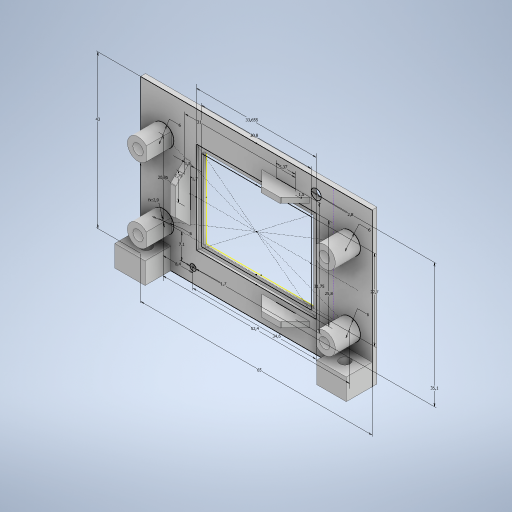
# Autodesk Inventor part: clamp
Saved by Autodesk Inventor 2024 (Build 280153000, 153)
## iProperties
Created: 2024-09-23
Part Number: clamp
Material: Generic
Document SubType Name: Modeling
Designer: PC
Density: 1 g/cm^3
Appearance: Default
Author: PC
Autodesk Inventor part; units mm, degrees
ref_plane "YZ Plane" through (0, 0, 0) normal (1, 0, 0) x (0, 1, 0)
ref_plane "XZ Plane" through (0, 0, 0) normal (0, 1, 0) x (-1, 0, 0)
ref_plane "XY Plane" through (0, 0, 0) normal (0, 0, 1) x (1, 0, 0)
sketch "Sketch1" plane through (0, 0, 0) normal (0, 0, 1) x (1, 0, 0)
  circle A0 centre (0, 0) radius 1.45
  line L0 (0, 0) -> (29.0858, 0) construction
  line L1 (0, 0) -> (0, 12.0151) construction
  circle A1 centre (52.4, 0) radius 1.45
  circle A2 centre (0, 20.95) radius 1.45
  circle A3 centre (52.4, 20.95) radius 1.45
  line L2 (9.3725, 23.375) -> (43.0275, 23.375)
  line L3 (43.0275, 23.375) -> (43.0275, -2.425)
  line L4 (43.0275, -2.425) -> (9.3725, -2.425)
  line L5 (9.3725, -2.425) -> (9.3725, 23.375)
  line L6 (0, 0) -> (52.4, 0) construction
  line L7 (0, 0) -> (0, 20.95) construction
  line L8 (31.8025, 26.35) -> (37.1725, 26.35)
  line L9 (37.1725, 26.35) -> (37.1725, 24.85)
  line L10 (37.1725, 24.85) -> (31.8025, 24.85)
  line L11 (31.8025, 24.85) -> (31.8025, 26.35)
  line L12 (0, 10.475) -> (54.8086, 10.475) construction
  line L13 (31.8025, -5.4) -> (37.1725, -5.4)
  line L14 (37.1725, -5.4) -> (37.1725, -3.9)
  line L15 (37.1725, -3.9) -> (31.8025, -3.9)
  line L16 (31.8025, -3.9) -> (31.8025, -5.4)
  line L17 (6.1725, 14.35) -> (7.6725, 14.35)
  line L18 (7.6725, 14.35) -> (7.6725, 6.6)
  line L19 (7.6725, 6.6) -> (6.1725, 6.6)
  line L20 (6.1725, 6.6) -> (6.1725, 14.35)
  line L21 (-6.3, 31.975) -> (58.7, 31.975)
  line L22 (58.7, 31.975) -> (58.7, -11.025)
  line L23 (58.7, -11.025) -> (-6.3, -11.025)
  line L24 (-6.3, -11.025) -> (-6.3, 31.975)
  line L25 (10.8, 21.825) -> (41.6, 21.825)
  line L26 (41.6, 21.825) -> (41.6, -0.875)
  line L27 (41.6, -0.875) -> (10.8, -0.875)
  line L28 (10.8, -0.875) -> (10.8, 21.825)
  line L29 (9.3725, -2.425) -> (43.0275, 23.375) construction
  line L30 (9.3725, 23.375) -> (43.0275, -2.425) construction
  circle A4 centre (0, 0) radius 3
  circle A5 centre (0, 20.95) radius 3
  circle A6 centre (52.4, 20.95) radius 3
  circle A7 centre (52.4, 0) radius 3
  line L31 (0, 0) -> (52.4, 20.95) construction
  line L32 (0, 20.95) -> (52.4, 0) construction
  circle A8 centre (8.4, -7.1) radius 0.85
  circle A9 centre (43, 28) radius 1.4
  point P0 (9.3725, 10.475)
  point P1 (26.2, 0)
  point P2 (26.2, -2.425)
  point P3 (7.6725, 10.475)
  point P4 (37.1725, 25.6)
  point P5 (26.2, 10.475)
  point P6 (26.2, 21.825)
  point P7 (26.2, 10.475)
  point P8 (41.6, 10.475)
  point P9 (-6.3, 10.475)
  point P10 (26.2, 31.975)
  dimension "d0" = 2.9
  dimension "d3" = 52.4
  dimension "d6" = 20.95
  dimension "d9" = 33.655
  dimension "d10" = 25.8
  dimension "d11" = 5.37
  dimension "d12" = 1.5
  dimension "d15" = 7.75
  dimension "d16" = 31.75
  dimension "d17" = 31
  dimension "d18" = 1.5
  dimension "d19" = 1.7
  dimension "d20" = 30.8
  dimension "d21" = 22.7
  dimension "d22" = 43
  dimension "d23" = 65
  dimension "d31" = 6
  dimension "d32" = 6
  dimension "d33" = 6
  dimension "d34" = 6
  dimension "d50" = 7.1
  dimension "d51" = 34.6
  dimension "d52" = 8.4
  dimension "d53" = 1.7
  dimension "d54" = 2.8
  dimension "d55" = 35.1
  constraints: 66 end point, 12 midpoint, 10 centre point, 10 parallel, 9 horizontal, 5 coincident, 5 perpendicular, 4 symmetric about line, 3 horizontal alignment, 3 vertical, 3 vertical alignment, 1 point on line, 6 other
  measures "d0" diameter of A0
  measures "d3" distance of L0.start L6.end
  measures "d6" distance of L0.start L7.end
  measures "d9" distance of L2.start L2.end
  measures "d10" distance of L2.end L3.end
  measures "d11" distance of L8.start L8.end
  measures "d12" distance of L8.end L9.end
  measures "d15" distance of L19.end L17.start
  measures "d16" distance between parallel lines of L13 L8
  measures "d17" distance from line of L20 point (37.173, 25.6)
  measures "d18" distance of L17.start L17.end
  measures "d19" distance between parallel lines of L5 L18
  measures "d20" distance of L25.start L25.end
  measures "d21" distance of L25.end L26.end
  measures "d22" distance of L23.end L21.start
  measures "d23" distance between parallel lines of L22 L24
  measures "d31" diameter of A4
  measures "d32" diameter of A5
  measures "d33" diameter of A6
  measures "d34" diameter of A7
  measures "d50" vertical distance of A8.centre point (0, 0)
  measures "d51" horizontal distance of A9.centre A8.centre
  measures "d52" horizontal distance of point (0, 0) A8.centre
  measures "d53" diameter of A8
  measures "d54" diameter of A9
  measures "d55" vertical distance of A8.centre A9.centre
extrude "Extrusion1" add sketch "Sketch1" against normal blind 1.4 contours L8 L9 L10 L11 | L16 L15 L14 L13 | L17 L18 L19 L20 | L21 L22 L23 L24 | A4 | A5 | A6 | A7 | A8 | A9
extrude "Extrusion2" add sketch "Sketch1" along normal blind 4.2 contours L8 L9 L10 L11 | L16 L15 L14 L13 | L17 L18 L19 L20
extrude "Extrusion3" add sketch "Sketch1" along normal blind 7 contours A4 | A5 | A6 | A7
sketch "Sketch3" plane through (0, 20.95, 7) normal (0, 0, 1) x (1, 0, 0)
  line L0 (2.3, 3.2266) -> (50.1, 3.2266)
  line L1 (50.1, 3.2266) -> (50.1, -23.7734)
  line L2 (50.1, -23.7734) -> (2.3, -23.7734)
  line L3 (2.3, -23.7734) -> (2.3, 3.2266)
  circle A0 centre (0, 0) radius 3 projected
  circle A1 centre (52.4, 0) radius 3 projected
  line L4 (2.3, -23.7734) -> (50.1, 3.2266) construction
  line L5 (2.3, 3.2266) -> (50.1, -23.7734) construction
  line L6 (9.3725, 2.425) -> (43.0275, 2.425) construction
  line L7 (4.5388, -3.9941) -> (9.4225, -3.9941)
  line L8 (9.4225, -3.9941) -> (9.4225, -17.6824)
  line L9 (9.4225, -17.6824) -> (4.5388, -17.6824)
  line L10 (4.5388, -17.6824) -> (4.5388, -3.9941)
  point P0 (0, -20.95)
  point P1 (26.2, -10.2734)
  point P2 (26.2, 2.425)
  point P3 (2.3, 1.9261)
  point P4 (2.3, -1.9261)
  point P5 (50.1, -1.9261)
  point P6 (50.1, 1.9261)
  dimension "d37" = 47.8
  dimension "d40" = 27
  constraints: 20 end point, 4 parallel, 2 horizontal, 2 midpoint, 2 perpendicular, 1 vertical alignment
  measures "d37" distance of L0.start L0.end
  measures "d40" distance between parallel lines of L2 L0
extrude "Extrusion4" cut sketch "Sketch3" against normal up to surface (7 mm away) contours L0 L1 A1 L2 L3 A0 | A0 L3 | L1 A1 picked at (2.4273, 0.4482) picked at (49.8935, -0.2303)
extrude "Extrusion5" add sketch "Sketch1" against normal blind 1.4 contours L2 L3 L4 L5
extrude "Extrusion6" cut sketch "Sketch1" against normal blind 0.7 contours L2 L3 L4 L5
sketch "Sketch5" plane through (0, 0, 0) normal (0, 0, 1) x (1, 0, 0)
  line L0 (58.7, -11.025) -> (-6.3, -11.025) construction
  line L1 (47.9657, -11.025) -> (47.9657, 31.975) construction
  line L2 (-6.3, 31.975) -> (58.7, 31.975) construction
  point P0 (0, 0)
  constraints: 2 end point, 2 point on line, 1 vertical
sketch "Sketch2" plane through (-6.3, -11.025, 0) normal (0, -1, 0) x (1, 0, 0)
  circle A0 centre (60.9, 3.5) radius 1.45
  circle A1 centre (5.1, 3.5) radius 1.5013
  line L0 (0, 0) -> (65, 0) projected
  line L1 (5.1, 3.5) -> (60.9, 3.5) construction
  line L2 (65, 0) -> (56.7123, 0)
  line L3 (56.7123, 0) -> (56.7123, 7.2261)
  line L4 (56.7123, 7.2261) -> (65, 7.2261)
  line L5 (65, 7.2261) -> (65, 0)
  line L6 (8.4882, 7.2261) -> (0, 7.2261)
  line L7 (0, 7.2261) -> (0, 0)
  line L8 (0, 0) -> (8.4882, 0)
  line L9 (8.4882, 0) -> (8.4882, 7.2261)
  point P0 (6.3, 0)
  point P1 (56.4, 7)
  dimension "d28" = 2.9
  dimension "d29" = 55.8
  dimension "d30" = 3.5
  dimension "d47" = 4.5
  constraints: 18 end point, 4 parallel, 3 horizontal, 2 centre point, 2 perpendicular, 1 point on line
  measures "d28" diameter of A0
  measures "d29" distance of L1.end L1.start
  measures "d30" distance from line of L0 L1.start
  measures "d47" horizontal distance of L1.end point (56.4, 7)
sketch "Sketch4" plane through (0, 0, -1.4) normal (0, 0, -1) x (-1, 0, 0)
  line L0 (-7.1929, 23.3228) -> (-45.2071, 23.3228)
  line L1 (-45.2071, 23.3228) -> (-45.2071, -2.3728)
  line L2 (-45.2071, -2.3728) -> (-7.1929, -2.3728)
  line L3 (-7.1929, -2.3728) -> (-7.1929, 23.3228)
  line L4 (-2.8715, 28.8309) -> (-49.5285, 28.8309)
  line L5 (-49.5285, 28.8309) -> (-49.5285, -7.8809)
  line L6 (-49.5285, -7.8809) -> (-2.8715, -7.8809)
  line L7 (-2.8715, -7.8809) -> (-2.8715, 28.8309)
  line L8 (-10.8, -0.875) -> (-41.6, -0.875) projected
  line L9 (-10.8, 21.825) -> (-10.8, -0.875) projected
  point P0 (0, 0)
  point P1 (-26.2, -2.3728)
  point P2 (-26.2, -0.875)
  point P3 (-10.8, 10.475)
  point P4 (-7.1929, 10.475)
  point P5 (-2.8715, 10.475)
  point P6 (-26.2, -7.8809)
  point P7 (-26.2, -0.875)
  constraints: 16 end point, 7 midpoint, 4 parallel, 3 vertical alignment, 2 horizontal, 2 horizontal alignment, 2 perpendicular
extrude "Extrusion7" add sketch "Sketch2" against normal blind 6
extrude "Extrusion8" cut sketch "Sketch1" against normal through all contours A8 | A9
chamfer "Chamfer1" distance 4 angle 45 6 edges at (6.9225, 14.35, 0) (6.9225, 6.6, 0) (31.8025, -4.65, 0) (37.1725, -4.65, 0) (37.1725, 25.6, 0) (31.8025, 25.6, 0)
equation "\"d0\" = m3"
equation "\"d28\" = m3"
equation "\"m3\" = 2.9"
body "Solid1"
